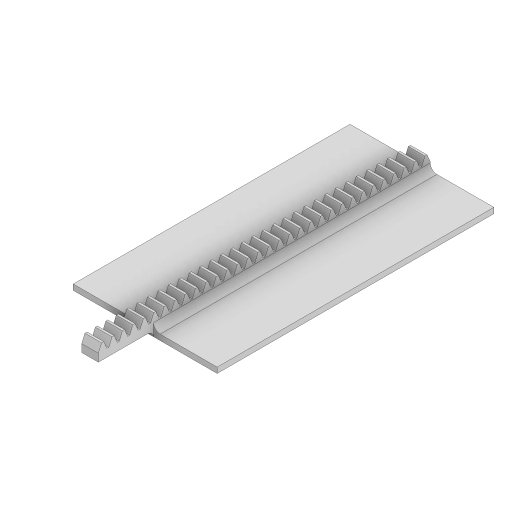
# Autodesk Inventor part: TAPA PRICIPAL CON CREMALLERA
Saved by Autodesk Inventor 2024 (Build 280153000, 153)
## iProperties
Created: 2024-06-13
Part Number: TAPA PRICIPAL CON CREMALLERA
Material: Generic
Document SubType Name: Modeling
Designer: Jhuliams
Density: 1 g/cm^3
Appearance: Default
Author: Jhuliams
Autodesk Inventor part; units mm, degrees
ref_plane "YZ Plane" through (0, 0, 0) normal (1, 0, 0) x (0, 1, 0)
ref_plane "XZ Plane" through (0, 0, 0) normal (0, 1, 0) x (-1, 0, 0)
ref_plane "XY Plane" through (0, 0, 0) normal (0, 0, 1) x (1, 0, 0)
sketch "Sketch4" plane through (0, 0, 0) normal (1, 0, 0) x (0, 1, 0)
  line L0 (0, -16.645) -> (0, -21.1217)
  line L1 (3, -17.923) -> (3, -19.8438)
  line L2 (3, -19.8438) -> (-3.75, -22.7192)
  line L3 (0, -21.1217) -> (0, -16.645)
  line L4 (0, -18.8834) -> (0.5045, -18.8834)
  line L5 (3, -17.923) -> (-3.75, -15.0476)
  line L6 (0, -7.2203) -> (0, -11.697)
  line L7 (3, -8.4983) -> (3, -10.419)
  line L8 (3, -10.419) -> (-3.75, -13.2945)
  line L9 (0, -11.697) -> (0, -7.2203)
  line L10 (0, -9.4587) -> (0.5045, -9.4587)
  line L11 (3, -8.4983) -> (-3.75, -5.6229)
  line L12 (0, 2.2044) -> (0, -2.2723)
  line L13 (3, 0.9264) -> (3, -0.9943)
  line L14 (3, -0.9943) -> (-3.75, -3.8698)
  line L15 (0, -2.2723) -> (0, 2.2044)
  line L16 (0, -0.034) -> (0.5045, -0.034)
  line L17 (3, 0.9264) -> (-3.75, 3.8018)
  line L18 (0, 11.6291) -> (0, 7.1524)
  line L19 (3, 10.3511) -> (3, 8.4304)
  line L20 (3, 8.4304) -> (-3.75, 5.5549)
  line L21 (0, 7.1524) -> (0, 11.6291)
  line L22 (0, 9.3907) -> (0.5045, 9.3907)
  line L23 (3, 10.3511) -> (-3.75, 13.2265)
  line L24 (0, 21.0538) -> (0, 16.5771)
  line L25 (3, 19.7758) -> (3, 17.8551)
  line L26 (3, 17.8551) -> (-3.75, 14.9796)
  line L27 (0, 16.5771) -> (0, 21.0538)
  line L28 (0, 18.8154) -> (0.5045, 18.8154)
  line L29 (3, 19.7758) -> (-3.75, 22.6512)
  line L30 (0, 30.4785) -> (0, 26.0018)
  line L31 (3, 29.2005) -> (3, 27.2797)
  line L32 (3, 27.2797) -> (-3.75, 24.4043)
  line L33 (0, 26.0018) -> (0, 30.4785)
  line L34 (0, 28.2401) -> (0.5045, 28.2401)
  line L35 (3, 29.2005) -> (-3.75, 32.0759)
  line L36 (0, 39.9032) -> (0, 35.4265)
  line L37 (3, 38.6252) -> (3, 36.7045)
  line L38 (3, 36.7045) -> (-3.75, 33.829)
  line L39 (0, 35.4265) -> (0, 39.9032)
  line L40 (0, 37.6648) -> (0.5045, 37.6648)
  line L41 (3, 38.6252) -> (-3.75, 41.5006)
  line L42 (0, 49.3279) -> (0, 44.8512)
  line L43 (3, 48.0499) -> (3, 46.1292)
  line L44 (3, 46.1292) -> (-3.75, 43.2537)
  line L45 (0, 44.8512) -> (0, 49.3279)
  line L46 (0, 47.0895) -> (0.5045, 47.0895)
  line L47 (3, 48.0499) -> (-3.75, 50.9253)
  line L48 (0, 58.7526) -> (0, 54.2759)
  line L49 (3, 57.4746) -> (3, 55.5539)
  line L50 (3, 55.5539) -> (-3.75, 52.6784)
  line L51 (0, 54.2759) -> (0, 58.7526)
  line L52 (0, 56.5142) -> (0.5045, 56.5142)
  line L53 (3, 57.4746) -> (-3.75, 60.35)
  line L54 (0, 68.1773) -> (0, 63.7006)
  line L55 (3, 66.8993) -> (3, 64.9785)
  line L56 (3, 64.9785) -> (-3.75, 62.1031)
  line L57 (0, 63.7006) -> (0, 68.1773)
  line L58 (0, 65.9389) -> (0.5045, 65.9389)
  line L59 (3, 66.8993) -> (-3.75, 69.7747)
  line L60 (0, 77.602) -> (0, 73.1253)
  line L61 (3, 76.324) -> (3, 74.4032)
  line L62 (3, 74.4032) -> (-3.75, 71.5278)
  line L63 (0, 73.1253) -> (0, 77.602)
  line L64 (0, 75.3636) -> (0.5045, 75.3636)
  line L65 (3, 76.324) -> (-3.75, 79.1994)
  line L66 (0, 87.0267) -> (0, 82.55)
  line L67 (3, 85.7487) -> (3, 83.828)
  line L68 (3, 83.828) -> (-3.75, 80.9525)
  line L69 (0, 82.55) -> (0, 87.0267)
  line L70 (0, 84.7883) -> (0.5045, 84.7883)
  line L71 (3, 85.7487) -> (-3.75, 88.6241)
  line L72 (0, 96.4514) -> (0, 91.9747)
  line L73 (3, 95.1734) -> (3, 93.2527)
  line L74 (3, 93.2527) -> (-3.75, 90.3772)
  line L75 (0, 91.9747) -> (0, 96.4514)
  line L76 (0, 94.213) -> (0.5045, 94.213)
  line L77 (3, 95.1734) -> (-3.75, 98.0488)
  line L78 (0, 105.8761) -> (0, 101.3994)
  line L79 (3, 104.5981) -> (3, 102.6774)
  line L80 (3, 102.6774) -> (-3.75, 99.8019)
  line L81 (0, 101.3994) -> (0, 105.8761)
  line L82 (0, 103.6377) -> (0.5045, 103.6377)
  line L83 (3, 104.5981) -> (-3.75, 107.4735)
  line L84 (0, 115.3008) -> (0, 110.8241)
  line L85 (3, 114.0228) -> (3, 112.1021)
  line L86 (3, 112.1021) -> (-3.75, 109.2266)
  line L87 (0, 110.8241) -> (0, 115.3008)
  line L88 (0, 113.0624) -> (0.5045, 113.0624)
  line L89 (3, 114.0228) -> (-3.75, 116.8982)
  line L90 (0, 124.7255) -> (0, 120.2488)
  line L91 (3, 123.4475) -> (3, 121.5268)
  line L92 (3, 121.5268) -> (-3.75, 118.6513)
  line L93 (0, 120.2488) -> (0, 124.7255)
  line L94 (0, 122.4871) -> (0.5045, 122.4871)
  line L95 (3, 123.4475) -> (-3.75, 126.3229)
  line L96 (0, 134.1502) -> (0, 129.6735)
  line L97 (3, 132.8722) -> (3, 130.9514)
  line L98 (3, 130.9514) -> (-3.75, 128.076)
  line L99 (0, 129.6735) -> (0, 134.1502)
  line L100 (0, 131.9118) -> (0.5045, 131.9118)
  line L101 (3, 132.8722) -> (-3.75, 135.7476)
  line L102 (0, 143.5749) -> (0, 139.0982)
  line L103 (3, 142.2969) -> (3, 140.3761)
  line L104 (3, 140.3761) -> (-3.75, 137.5007)
  line L105 (0, 139.0982) -> (0, 143.5749)
  line L106 (0, 141.3365) -> (0.5045, 141.3365)
  line L107 (3, 142.2969) -> (-3.75, 145.1723)
  line L108 (0, 152.9996) -> (0, 148.5229)
  line L109 (3, 151.7216) -> (3, 149.8008)
  line L110 (3, 149.8008) -> (-3.75, 146.9254)
  line L111 (0, 148.5229) -> (0, 152.9996)
  line L112 (0, 150.7612) -> (0.5045, 150.7612)
  line L113 (3, 151.7216) -> (-3.75, 154.597)
  line L114 (0, 162.4243) -> (0, 157.9476)
  line L115 (3, 161.1463) -> (3, 159.2255)
  line L116 (3, 159.2255) -> (-3.75, 156.3501)
  line L117 (0, 157.9476) -> (0, 162.4243)
  line L118 (0, 160.1859) -> (0.5045, 160.1859)
  line L119 (3, 161.1463) -> (-3.75, 164.0217)
  line L120 (0, 171.849) -> (0, 167.3723)
  line L121 (3, 170.571) -> (3, 168.6502)
  line L122 (3, 168.6502) -> (-3.75, 165.7748)
  line L123 (0, 167.3723) -> (0, 171.849)
  line L124 (0, 169.6106) -> (0.5045, 169.6106)
  line L125 (3, 170.571) -> (-3.75, 173.4464)
  line L126 (0, 181.2737) -> (0, 176.797)
  line L127 (3, 179.9957) -> (3, 178.075)
  line L128 (3, 178.075) -> (-3.75, 175.1995)
  line L129 (0, 176.797) -> (0, 181.2737)
  line L130 (0, 179.0353) -> (0.5045, 179.0353)
  line L131 (3, 179.9957) -> (-3.75, 182.8711)
  line L132 (0, 190.6984) -> (0, 186.2217)
  line L133 (3, 189.4204) -> (3, 187.4997)
  line L134 (3, 187.4997) -> (-3.75, 184.6242)
  line L135 (0, 186.2217) -> (0, 190.6984)
  line L136 (0, 188.46) -> (0.5045, 188.46)
  line L137 (3, 189.4204) -> (-3.75, 192.2958)
  line L138 (0, 200.1231) -> (0, 195.6464)
  line L139 (3, 198.8451) -> (3, 196.9244)
  line L140 (3, 196.9244) -> (-3.75, 194.0489)
  line L141 (0, 195.6464) -> (0, 200.1231)
  line L142 (0, 197.8847) -> (0.5045, 197.8847)
  line L143 (3, 198.8451) -> (-3.75, 201.7205)
  line L144 (0, 209.5478) -> (0, 205.0711)
  line L145 (3, 208.2698) -> (3, 206.3491)
  line L146 (3, 206.3491) -> (-3.75, 203.4736)
  line L147 (0, 205.0711) -> (0, 209.5478)
  line L148 (0, 207.3094) -> (0.5045, 207.3094)
  line L149 (3, 208.2698) -> (-3.75, 211.1452)
  line L150 (0, 218.9725) -> (0, 214.4958)
  line L151 (3, 217.6945) -> (3, 215.7738)
  line L152 (3, 215.7738) -> (-3.75, 212.8983)
  line L153 (0, 214.4958) -> (0, 218.9725)
  line L154 (0, 216.7341) -> (0.5045, 216.7341)
  line L155 (3, 217.6945) -> (-3.75, 220.5699)
  line L156 (0, 228.3972) -> (0, 223.9205)
  line L157 (3, 227.1192) -> (3, 225.1985)
  line L158 (3, 225.1985) -> (-3.75, 222.323)
  line L159 (0, 223.9205) -> (0, 228.3972)
  line L160 (0, 226.1588) -> (0.5045, 226.1588)
  line L161 (3, 227.1192) -> (-3.75, 229.9946)
  line L162 (0, 237.8219) -> (0, 233.3452)
  line L163 (3, 236.5439) -> (3, 234.6232)
  line L164 (3, 234.6232) -> (-3.75, 231.7477)
  line L165 (0, 233.3452) -> (0, 237.8219)
  line L166 (0, 235.5835) -> (0.5045, 235.5835)
  line L167 (3, 236.5439) -> (-3.75, 239.4193)
  line L168 (0, 247.2466) -> (0, 242.7699)
  line L169 (3, 245.9686) -> (3, 244.0479)
  line L170 (3, 244.0479) -> (-3.75, 241.1724)
  line L171 (0, 242.7699) -> (0, 247.2466)
  line L172 (0, 245.0082) -> (0.5045, 245.0082)
  line L173 (3, 245.9686) -> (-3.75, 248.844)
  line L174 (0, 256.6713) -> (0, 252.1946)
  line L175 (3, 255.3933) -> (3, 253.4726)
  line L176 (3, 253.4726) -> (-3.75, 250.5971)
  line L177 (0, 252.1946) -> (0, 256.6713)
  line L178 (0, 254.4329) -> (0.5045, 254.4329)
  line L179 (3, 255.3933) -> (-3.75, 258.2687)
  line L180 (0, 266.096) -> (0, 261.6193)
  line L181 (3, 264.818) -> (3, 262.8972)
  line L182 (3, 262.8972) -> (-3.75, 260.0218)
  line L183 (0, 261.6193) -> (0, 266.096)
  line L184 (0, 263.8576) -> (0.5045, 263.8576)
  line L185 (3, 264.818) -> (-3.75, 267.6934)
  line L186 (0, 275.5207) -> (0, 271.044)
  line L187 (3, 274.2427) -> (3, 272.322)
  line L188 (3, 272.322) -> (-3.75, 269.4465)
  line L189 (0, 271.044) -> (0, 275.5207)
  line L190 (0, 273.2823) -> (0.5045, 273.2823)
  line L191 (3, 274.2427) -> (-3.75, 277.1181)
  line L192 (-3.75, 277.1181) -> (-10.75, 277.1181)
  line L193 (-10.75, 277.1181) -> (-10.75, -22.7192)
  line L194 (-10.75, -22.7192) -> (-3.75, -22.7192)
  line L195 (-3.75, -22.7192) -> (-3.75, 277.1181)
  point P0 (-3.75, -22.7192)
  point P1 (-3.75, -13.2945)
  point P2 (-3.75, -3.8698)
  point P3 (-3.75, 5.5549)
  point P4 (-3.75, 14.9796)
  point P5 (-3.75, 24.4043)
  point P6 (-3.75, 33.829)
  point P7 (-3.75, 43.2537)
  point P8 (-3.75, 52.6784)
  point P9 (-3.75, 62.1031)
  point P10 (-3.75, 71.5278)
  point P11 (-3.75, 80.9525)
  point P12 (-3.75, 90.3772)
  point P13 (-3.75, 99.8019)
  point P14 (-3.75, 109.2266)
  point P15 (-3.75, 118.6513)
  point P16 (-3.75, 128.076)
  point P17 (-3.75, 137.5007)
  point P18 (-3.75, 146.9254)
  point P19 (-3.75, 156.3501)
  point P20 (-3.75, 165.7748)
  point P21 (-3.75, 175.1995)
  point P22 (-3.75, 184.6242)
  point P23 (-3.75, 194.0489)
  point P24 (-3.75, 203.4736)
  point P25 (-3.75, 212.8983)
  point P26 (-3.75, 222.323)
  point P27 (-3.75, 231.7477)
  point P28 (-3.75, 241.1724)
  point P29 (-3.75, 250.5971)
  point P30 (-3.75, 260.0218)
  point P31 (-3.75, 269.4465)
  dimension "d53" = 3
  dimension "d56" = 4.4767
  dimension "d61" = 9.4247
  dimension "d66" = 7
  constraints: 390 end point, 64 point on line, 3 vertical, 2 horizontal, 2 parallel, 1 collinear, 1 midpoint, 1 perpendicular, 1 symmetric about line, 436 other
  measures "d53" distance between parallel lines of L0 L1
  measures "d56" distance of L0.start L0.end
  measures "d61" distance of L0.start L6.start
  measures "d66" distance of L194.end L193.end
extrude "Extrusion2" add sketch "Sketch4" along normal blind 15
sketch "Sketch7" plane through (0, -10.75, -22.7192) normal (0, -1, 0) x (1, 0, 0)
  line L0 (0, 0) -> (0, 2.8755) projected
  line L1 (0, 0) -> (7.5, 0)
  line L2 (0, 0) -> (15, 0) projected
  line L3 (72.5, 250) -> (-57.5, 250)
  line L4 (-57.5, 250) -> (-57.5, -250)
  line L5 (-57.5, -250) -> (72.5, -250)
  line L6 (72.5, -250) -> (72.5, 250)
  line L7 (72.5, 250) -> (-57.5, -250) construction
  line L8 (-57.5, 250) -> (72.5, -250) construction
  line L9 (72.5, 0) -> (-57.5, 0)
  point P0 (0, 22.7192)
  dimension "d67" = 7.5
  dimension "d68" = 130
  dimension "d69" = 500
  constraints: 16 end point, 5 midpoint, 2 parallel, 1 horizontal, 1 perpendicular
  measures "d67" distance of L0.start L1.end
  measures "d68" distance of L5.end L4.end
  measures "d69" distance of L4.end L3.end
extrude "Extrusion5" add sketch "Sketch7" along normal blind 5 contours L9 L4 L3 L6 L2 L1
fillet "Fillet1" radius 6 2 edges at (15, -10.75, 102.2808) (0, -10.75, 102.2808)
fillet "Fillet2" radius 6 1 edges at (7.5, -10.75, 227.2808)
body "Solid2"
